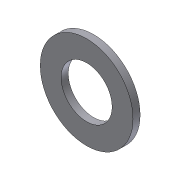
# Autodesk Inventor part: NAS620-C4L / MCMASTER-CARR 90945A710
Saved by Autodesk Inventor 2014 SP1 (Build 180222100, 222)
## iProperties
Created: 2009-09-14
Part Number: NAS620-C4L / MCMASTER-CARR 90945A710
Document SubType Name: Modeling
Designer: Robert Davis
Density: 8.08 g/cm^3
Material: Stainless Steel
Mass: 0.0506752 g
Surface Area: 0.413717 cm^2
Volume: 0.00627168 cm^3
Description: WASHER, #4 THIN
Appearance: Steel
Author: Robert Davis
Autodesk Inventor part; units mm, degrees
ref_plane "YZ Plane" through (0, 0, 0) normal (1, 0, 0) x (0, 1, 0)
ref_plane "XZ Plane" through (0, 0, 0) normal (0, 1, 0) x (-1, 0, 0)
ref_plane "XY Plane" through (0, 0, 0) normal (0, 0, 1) x (1, 0, 0)
sketch "Sketch1" plane through (0, 0, 0) normal (0, 0, 1) x (1, 0, 0)
  circle A0 centre (0, 0) radius 1.4605
  circle A1 centre (0, 0) radius 2.6543
  dimension "d0" = 2.921
  dimension "d1" = 5.3086
  constraints: 2 centre point, 1 coincident
  measures "d0" diameter of A0
  measures "d1" diameter of A1
extrude "Extrusion1" add sketch "Sketch1" along normal mid plane 0.4064
body "Solid1"
